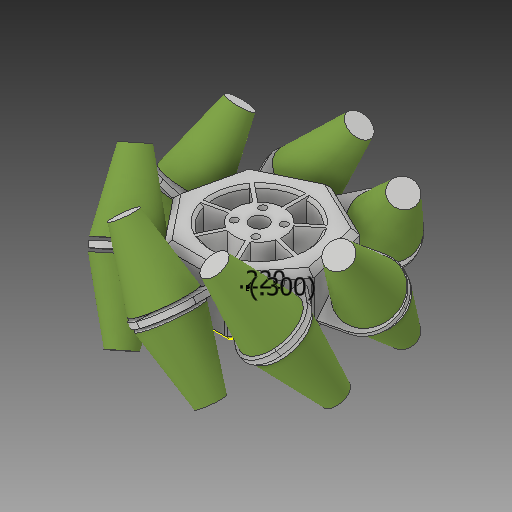
# Autodesk Inventor part: Mecanum Wheel Plastic Base
Saved by Autodesk Inventor 2017 (Build 210142000, 142)
## iProperties
Created: 2017-10-03
Part Number: Mecanum Wheel Plastic Base
Material: Generic
Document SubType Name: Modeling
Designer: 308075
Density: 1 g/cm^3
Appearance: Default
Author: 308075
Autodesk Inventor part; units mm, degrees
ref_plane "YZ Plane" through (0, 0, 0) normal (1, 0, 0) x (0, 1, 0)
sketch "Sketch1" plane through (0, 0, 0) normal (0, 1, 0) x (-1, 0, 0)
  circle A0 centre (0, 0) radius 8.89
  arc A1 (0, -8.89) -> (5.5337, -6.9577) centre (0, 0) ccw
  arc A2 (0, -8.89) -> (5.5337, -6.9577) centre (0, 0) ccw
  arc A3 (0.0644, 8.8898) -> (0, 8.89) centre (0, 0) ccw
  arc A4 (8.8891, -0.1295) -> (8.89, -0.0116) centre (0, 0) ccw
  arc A5 (-8.0046, 3.8677) -> (0, -8.89) centre (0, 0) ccw
  arc A6 (-8.8898, 0.0606) -> (-3.6012, -8.1279) centre (0, 0) ccw
  arc A7 (0, -8.89) -> (8.89, -0.0116) centre (0, 0) ccw
  arc A8 (5.5519, 6.9432) -> (-4.757, 7.5102) centre (0, 0) ccw
  arc A9 (8.89, -0.0116) -> (0, 8.89) centre (0, 0) ccw
  line L0 (-13.9547, 28.8724) -> (13.8727, 28.9118)
  line L1 (13.8727, 28.9118) -> (31.2537, 7.1801)
  line L2 (31.2537, 7.1801) -> (25.1, -19.9584)
  line L3 (25.1, -19.9584) -> (0.0455, -32.0678)
  line L4 (0.0455, -32.0678) -> (-25.0433, -20.0295)
  line L5 (-25.0433, -20.0295) -> (-31.2739, 7.0914)
  line L6 (-31.2739, 7.0914) -> (-13.9547, 28.8724)
  circle A10 centre (0, 0) radius 20.32
  arc A11 (0.0455, 28.9118) -> (0.0098, 28.8922) centre (5.5387, 18.8884) ccw
  line L7 (0, -20.32) -> (0, -20.32)
  line L8 (-1.27, -8.8308) -> (1.27, -8.8308)
  line L9 (1.27, -8.8308) -> (1.27, -20.2803)
  line L10 (1.27, -20.2803) -> (-1.27, -20.2803)
  line L11 (-1.27, -20.2803) -> (-1.27, -8.8308)
  line L12 (-1.27, -8.8308) -> (1.27, -20.2803) construction
  line L13 (1.27, -8.8308) -> (-1.27, -20.2803) construction
  point P0 (0, -14.2762)
  point P1 (0, -14.5556)
  dimension "d1" = 17.78
  dimension "d6" = 60.96
  dimension "d23" = 40.64
  dimension "d24" = 11.43
  dimension "d25" = 2.54
  constraints: 30 point on circle, 28 end point, 13 coincident, 12 centre point, 2 horizontal, 2 midpoint, 2 parallel, 1 perpendicular, 1 point on line, 15 other
  measures "d1" diameter of A0
  measures "d6" distance from line of L0 L3.end
  measures "d23" diameter of A10
  measures "d24" radial gap between concentric circles of A10 A5
  measures "d25" distance of L9.end L10.end
extrude "Extrusion2" add sketch "Sketch1" along normal blind 25.4
sketch "Sketch8" plane through (0, 25.4, 0) normal (0, 1, 0) x (1, 0, 0)
  circle A0 centre (0, 0) radius 8.89
  circle A1 centre (0, 0) radius 3.81
  dimension "d30" = 17.78
  dimension "d31" = 7.62
  constraints: 2 centre point, 2 coincident
  measures "d30" diameter of A0
  measures "d31" diameter of A1
extrude "Extrusion3" add sketch "Sketch8" against normal blind 25.4
sketch "Sketch9" plane through (0, 25.4, 0) normal (0, 1, 0) x (1, 0, 0)
  circle A0 centre (0, 0) radius 20.32 projected
  circle A1 centre (0, 0) radius 8.89 projected
  circle A2 centre (0, 0) radius 20.32 projected
  line L0 (0, 8.89) -> (0, 20.32)
  line L1 (-0.9738, -0.6493) -> (0.9738, -0.6493)
  line L2 (0.9738, -0.6493) -> (0.9738, 0.6493)
  line L3 (0.9738, 0.6493) -> (-0.9738, 0.6493)
  line L4 (-0.9738, 0.6493) -> (-0.9738, -0.6493)
  line L5 (-0.9738, -0.6493) -> (0.9738, 0.6493) construction
  line L6 (0.9738, -0.6493) -> (-0.9738, 0.6493) construction
  line L7 (0, 0) -> (0.9217, 0)
  line L8 (0.7953, 20.5703) -> (-0.7953, 20.5703)
  line L9 (-0.7953, 20.5703) -> (-0.7953, 8.6397)
  line L10 (-0.7953, 8.6397) -> (0.7953, 8.6397)
  line L11 (0.7953, 8.6397) -> (0.7953, 20.5703)
  line L12 (0.7953, 20.5703) -> (-0.7953, 8.6397) construction
  line L13 (-0.7953, 20.5703) -> (0.7953, 8.6397) construction
  point P0 (0, 14.605)
  dimension "d43" = 5.715
  dimension "d44" = 1.2986
  dimension "d45" = 1.9476
  dimension "d46" = 90
  constraints: 28 end point, 5 midpoint, 4 parallel, 3 perpendicular, 3 vertical alignment, 2 horizontal, 3 other
  measures "d43" distance of L0.start point (0, 14.605)
  measures "d44" distance of L1.end L2.end
  measures "d45" distance of L2.end L3.end
  measures "d46" angle of L7 L0
extrude "Extrusion4" add sketch "Sketch9" against normal blind 25.4 contours L11 A1 L0 A0 | A0 L9 L8 L11 | A0 L0 A1 L9 | L11 L10 L9 A1 picked at (0, 8.7231)
pattern_circular "Circular Pattern1" count 7 over 360 about axis through (0, 25.4, 0) along (0, -1, 0) of "Extrusion4"
sketch "Sketch10" plane through (-0.0455, 0, -32.0678) normal (0.4326053, 0, -0.9015834) x (-0.9015834, 0, -0.4326053)
  point P0 (-13.9137, 0)
chamfer "Chamfer1" distance 2.54 angle 45 14 edges at (12.4989, 25.4, -26.0487) (-12.5727, 25.4, -26.0131) (-28.1768, 25.4, -6.3891) (-22.5632, 25.4, 18.046) (0.041, 25.4, 28.8921) (22.6143, 25.4, 17.9819) (28.1586, 25.4, -6.4691) (12.4989, 0, -26.0487) (-12.5727, 0, -26.0131) (-28.1768, 0, -6.3891) (-22.5632, 0, 18.046) (0.041, 0, 28.8921) (22.6143, 0, 17.9819) (28.1586, 0, -6.4691)
chamfer "Chamfer2" distance 1.27 angle 45 7 edges at (-19.8105, 0, -4.5216) (-15.8868, 0, 12.6693) (0, 0, 20.32) (15.8868, 0, 12.6693) (19.8105, 0, -4.5216) (8.8165, 0, -18.3077) (-8.8165, 0, -18.3077)
chamfer "Chamfer3" distance 1.27 angle 45 7 edges at (-8.8165, 25.4, -18.3077) (-19.8105, 25.4, -4.5216) (8.8165, 25.4, -18.3077) (19.8105, 25.4, -4.5216) (15.8868, 25.4, 12.6693) (0, 25.4, 20.32) (-15.8868, 25.4, 12.6693)
sketch "Sketch11" plane through (-25.1, 2.54, -19.9584) normal (-0.4351614, 0, -0.9003525) x (-0.9003525, 0, 0.4351614)
  line L0 (0, 0) -> (0, 20.32) projected
  line L1 (-27.824, 0.0599) -> (0, 20.32) construction
  line L2 (-27.8274, 0) -> (-27.8274, 20.32) projected
  line L3 (0, 0) -> (-27.8274, 20.32) construction
  line L4 (-13.9137, 0) -> (-13.9137, 20.32) construction
  line L5 (-13.9137, 0) -> (-13.9137, 20.32)
  line L6 (0.119, 10.16) -> (-27.8274, 10.16) construction
  line L7 (-13.9137, 10.16) -> (-25.2207, 1.9555) construction
  line L8 (-13.9137, 10.16) -> (-2.6204, 18.3833) construction
  line L9 (-13.9137, 10.16) -> (-12.8881, 9.411) construction
  line L10 (-13.9137, 10.16) -> (-14.9394, 10.909) construction
  line L11 (-14.9394, 10.909) -> (-3.3322, 19.3608)
  line L12 (-14.9394, 10.909) -> (-25.9499, 2.9196)
  line L13 (-12.8881, 9.411) -> (-24.5304, 0.9632)
  line L14 (-12.8881, 9.411) -> (-1.8905, 17.419)
  line L15 (-1.8905, 17.419) -> (-3.3322, 19.3608)
  line L16 (-24.5304, 0.9632) -> (-25.9499, 2.9196)
  point P0 (-13.9137, -2.54)
  dimension "d61" = 13.97
  dimension "d62" = 13.97
  dimension "d64" = 1.27
  dimension "d65" = 1.27
  constraints: 28 end point, 4 parallel, 4 point on line, 2 midpoint, 1 collinear, 1 horizontal, 1 perpendicular
  measures "d61" distance of L7.start L7.end
  measures "d62" distance of L7.start L8.end
  measures "d64" distance of L7.start L9.end
  measures "d65" distance of L7.start L10.end
fillet "Fillet1" radius 1.27 7 edges at (-0.0455, 12.7, -32.0678) (25.0433, 12.7, -20.0295) (31.2739, 12.7, 7.0914) (13.9547, 12.7, 28.8724) (-13.8727, 12.7, 28.9118) (-31.2537, 12.7, 7.1801) (-25.1, 12.7, -19.9584)
extrude "Extrusion6" add sketch "Sketch11" along normal blind 25.4
fillet "Fillet4" radius 13.97 2 edges at (-13.4281, 4.4814, -53.8109) (-33.802, 20.9299, -43.9637)
sketch "Sketch16" plane through (-23.3979, 19.959, -20.7811) normal (-0.5299804, -0.8083978, 0.2561519) x (0.7278429, -0.5886366, -0.3517835)
  line L0 (14.8742, -13.97) -> (12.3342, -13.97)
  line L1 (12.3342, -13.97) -> (12.3342, -11.43)
  line L2 (12.3342, -11.43) -> (14.8742, -11.43)
  line L3 (14.8742, -11.43) -> (14.8742, -13.97)
  line L4 (13.6042, 0) -> (13.6042, -25.4) projected
  line L5 (14.8742, -13.97) -> (12.3342, -11.43) construction
  line L6 (12.3342, -13.97) -> (14.8742, -11.43) construction
  point P0 (21.4681, 28.8921)
  point P1 (13.6042, -12.7)
  dimension "d80" = 2.54
  dimension "d81" = 2.54
  constraints: 12 end point, 3 midpoint, 2 parallel, 1 horizontal, 1 perpendicular
  measures "d80" distance of L1.end L2.end
  measures "d81" distance of L0.end L1.end
extrude "Extrusion7" add sketch "Sketch16" along normal blind 1.27
ref_plane "Work Plane2" through (-40.2248, -5.7077, -12.6482) normal (-0.5299804, -0.8083978, 0.2561519) x (0.7278429, -0.5886366, -0.3517835)
sketch "Sketch17" plane through (-40.2248, -5.7077, -12.6482) normal (-0.5299804, -0.8083978, 0.2561519) x (0.7278429, -0.5886366, -0.3517835)
  line L0 (13.6042, -11.43) -> (13.6042, -13.97) projected
  circle A0 centre (13.6042, -12.7) radius 5.715
  point P0 (21.4681, 28.8921)
  dimension "d85" = 11.43
  constraints: 1 centre point, 1 midpoint
  measures "d85" diameter of A0
sketch "Sketch18" plane through (-24.071, 18.9323, -20.4558) normal (-0.5299804, -0.8083978, 0.2561519) x (0.7278429, -0.5886366, -0.3517835)
  line L0 (13.6042, -11.43) -> (13.6042, -13.97) projected
  circle A0 centre (13.6042, -12.7) radius 12.7
  point P0 (21.4681, 28.8921)
  dimension "d86" = 25.4
  constraints: 1 centre point, 1 midpoint
  measures "d86" diameter of A0
loft "Loft1" add profiles "Sketch18", "Sketch17"
ref_plane "Work Plane3" through (-12.8572, 12.9292, -25.8756) normal (-0.5287712, -0.809374, 0.2555675) x (0.7287219, -0.5872936, -0.3522083)
mirror "Mirror1" about plane through (-12.8572, 12.9292, -25.8756) normal (-0.5287712, -0.809374, 0.2555675) of "Loft1"
pattern_circular "Circular Pattern4" count 7 over 360 about axis through (0, 25.4, 0) along (0, -1, 0) of "Loft1", "Extrusion6", "Fillet4", "Mirror1"
sketch "Sketch19" plane through (0, 0, 0) normal (0, -1, 0) x (1, 0, 0)
  line L0 (-16.3724, -14.0738) -> (-6.4267, -6.1424) projected
  arc A0 (-6.4267, -6.1424) -> (-0.7953, -8.8544) centre (0, 0) ccw projected
  line L1 (-0.7953, -21.5753) -> (-0.7953, -8.8544) projected
  arc A1 (-16.3724, -14.0738) -> (-0.7953, -21.5753) centre (0, 0) ccw projected
  line L2 (0.7953, -21.5753) -> (0.7953, -8.8544) projected
  arc A2 (0.7953, -8.8544) -> (6.4267, -6.1424) centre (0, 0) ccw projected
  line L3 (16.3724, -14.0738) -> (6.4267, -6.1424) projected
  arc A3 (0.7953, -21.5753) -> (16.3724, -14.0738) centre (0, 0) ccw projected
  line L4 (17.3642, -12.8302) -> (7.4185, -4.8988) projected
  arc A4 (7.4185, -4.8988) -> (8.8093, 1.1949) centre (0, 0) ccw projected
  line L5 (21.2114, 4.0256) -> (8.8093, 1.1949) projected
  arc A5 (17.3642, -12.8302) -> (21.2114, 4.0256) centre (0, 0) ccw projected
  line L6 (20.8574, 5.5764) -> (8.4554, 2.7457) projected
  arc A6 (8.4554, 2.7457) -> (4.5583, 7.6324) centre (0, 0) ccw projected
  line L7 (10.0778, 19.0936) -> (4.5583, 7.6324) projected
  arc A7 (20.8574, 5.5764) -> (10.0778, 19.0936) centre (0, 0) ccw projected
  line L8 (8.6446, 19.7838) -> (3.1252, 8.3226) projected
  arc A8 (3.1252, 8.3226) -> (-3.1252, 8.3226) centre (0, 0) ccw projected
  line L9 (-8.6446, 19.7838) -> (-3.1252, 8.3226) projected
  arc A9 (8.6446, 19.7838) -> (-8.6446, 19.7838) centre (0, 0) ccw projected
  line L10 (-10.0778, 19.0936) -> (-4.5583, 7.6324) projected
  arc A10 (-4.5583, 7.6324) -> (-8.4554, 2.7457) centre (0, 0) ccw projected
  line L11 (-20.8574, 5.5764) -> (-8.4554, 2.7457) projected
  arc A11 (-10.0778, 19.0936) -> (-20.8574, 5.5764) centre (0, 0) ccw projected
  line L12 (-21.2114, 4.0256) -> (-8.8093, 1.1949) projected
  arc A12 (-8.8093, 1.1949) -> (-7.4185, -4.8988) centre (0, 0) ccw projected
  line L13 (-17.3642, -12.8302) -> (-7.4185, -4.8988) projected
  arc A13 (-21.2114, 4.0256) -> (-17.3642, -12.8302) centre (0, 0) ccw projected
  circle A14 centre (0, 0) radius 3.81 projected
  line L14 (-12.6531, 26.3701) -> (12.7279, 26.3341) projected
  line L15 (-28.5061, 6.5489) -> (-12.6531, 26.3701) projected
  line L16 (-22.8934, -18.2038) -> (-28.5061, 6.5489) projected
  line L17 (-0.0415, -29.2486) -> (-22.8934, -18.2038) projected
  line L18 (22.8416, -18.2687) -> (-0.0415, -29.2486) projected
  line L19 (28.5245, 6.468) -> (22.8416, -18.2687) projected
  line L20 (12.7279, 26.3341) -> (28.5245, 6.468) projected
  line L21 (0, 0) -> (0, -1.6432)
  point P0 (-0.0079, -5.5821)
  dimension "d98" = 7.62
  dimension "d99" = 5.582
  constraints: 2 end point, 1 vertical
  measures "d98" diameter of A14
  measures "d99" distance of L21.start point (-0.008, -5.582)
sketch "Sketch20" plane through (0, 25.4, 0) normal (0, 1, 0) x (1, 0, 0)
  arc A0 (7.3557, 3.532) -> (5.4218, 6.098) centre (6.3887, 4.815) ccw projected
  arc A1 (5.4218, 6.098) -> (7.3557, 3.532) centre (6.3887, 4.815) ccw projected
  arc A2 (-3.8481, 5.1057) -> (-5.782, 7.6717) centre (-4.815, 6.3887) ccw projected
  arc A3 (-5.782, 7.6717) -> (-3.8481, 5.1057) centre (-4.815, 6.3887) ccw projected
  arc A4 (1.567, -2.0791) -> (-1.567, 2.0791) centre (0, 0) ccw projected
  arc A5 (-1.567, 2.0791) -> (1.567, -2.0791) centre (0, 0) ccw projected
  arc A6 (5.782, -7.6717) -> (3.8481, -5.1057) centre (4.815, -6.3887) ccw projected
  arc A7 (3.8481, -5.1057) -> (5.782, -7.6717) centre (4.815, -6.3887) ccw projected
  arc A8 (-5.4218, -6.098) -> (-7.3557, -3.532) centre (-6.3887, -4.815) ccw projected
  arc A9 (-7.3557, -3.532) -> (-5.4218, -6.098) centre (-6.3887, -4.815) ccw projected
  arc A10 (-6.6207, 8.7845) -> (6.6207, -8.7845) centre (0, 0) ccw projected
  arc A11 (6.6207, -8.7845) -> (-6.6207, 8.7845) centre (0, 0) ccw projected
  circle A12 centre (0, 0) radius 3.81
  point P0 (0, 0)
  constraints: 1 centre point, 1 coincident
extrude "Extrusion8" add sketch "Sketch20" against normal blind 25.4 contours A11 A10
sketch "Sketch21" plane through (0, 25.4, 0) normal (0, 1, 0) x (1, 0, 0)
  arc A0 (7.3557, 3.532) -> (5.4218, 6.098) centre (6.3887, 4.815) ccw projected
  arc A1 (5.4218, 6.098) -> (7.3557, 3.532) centre (6.3887, 4.815) ccw projected
  arc A2 (-3.8481, 5.1057) -> (-5.782, 7.6717) centre (-4.815, 6.3887) ccw projected
  arc A3 (-5.782, 7.6717) -> (-3.8481, 5.1057) centre (-4.815, 6.3887) ccw projected
  arc A4 (1.567, -2.0791) -> (-1.567, 2.0791) centre (0, 0) ccw projected
  arc A5 (-1.567, 2.0791) -> (1.567, -2.0791) centre (0, 0) ccw projected
  arc A6 (5.782, -7.6717) -> (3.8481, -5.1057) centre (4.815, -6.3887) ccw projected
  arc A7 (3.8481, -5.1057) -> (5.782, -7.6717) centre (4.815, -6.3887) ccw projected
  arc A8 (-5.4218, -6.098) -> (-7.3557, -3.532) centre (-6.3887, -4.815) ccw projected
  arc A9 (-7.3557, -3.532) -> (-5.4218, -6.098) centre (-6.3887, -4.815) ccw projected
  arc A10 (-6.6207, 8.7845) -> (6.6207, -8.7845) centre (0, 0) ccw projected
  arc A11 (6.6207, -8.7845) -> (-6.6207, 8.7845) centre (0, 0) ccw projected
  point P0 (0, 0)
extrude "Extrusion9" cut sketch "Sketch21" against normal blind 25.4 contours A1 A0 | A3 A2 | A7 A6 | A9 A8
body "Solid2"
